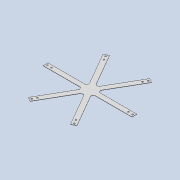
# Autodesk Inventor part: release_layer
Saved by Autodesk Inventor 2020 (Build 240168000, 168)
## iProperties
Created: 2021-10-03
Part Number: release_layer
Material: Generic
Document SubType Name: Modeling
Designer: Shuang Peng
Density: 1 g/cm^3
Appearance: Default
Author: Shuang Peng
Autodesk Inventor part; units mm, degrees
ref_plane "YZ Plane" through (0, 0, 0) normal (1, 0, 0) x (0, 1, 0)
ref_plane "XZ Plane" through (0, 0, 0) normal (0, 1, 0) x (-1, 0, 0)
ref_plane "XY Plane" through (0, 0, 0) normal (0, 0, 1) x (1, 0, 0)
sketch "Sketch1" plane through (0, 0, 0) normal (0, 1, 0) x (-1, 0, 0)
  line L0 (0, 0) -> (100, 0)
  line L1 (100, 0) -> (100, -100)
  line L2 (100, -100) -> (0, -100)
  line L3 (0, -100) -> (0, 0)
  dimension "d0" = 100
  dimension "d1" = 100
  constraints: 8 end point, 2 parallel, 1 horizontal, 1 perpendicular
  measures "d0" distance of L1.end L2.end
  measures "d1" distance of L0.end L1.end
extrude "Extrusion1" add sketch "Sketch1" along normal blind 0.2
sketch "Sketch2" plane through (0, 0.2, 0) normal (0, 1, 0) x (1, 0, 0)
  line L0 (-100, 0) -> (0, 0) projected
  line L1 (0, 0) -> (0, 50)
  line L2 (0, 50) -> (-50, 50)
  circle A0 centre (-50, 50) radius 6
  line L3 (-50, 50) -> (-77, 50)
  line L4 (-77, 48) -> (-77, 52)
  line L5 (-77, 52) -> (-50, 52)
  line L6 (-50, 52) -> (-50, 48)
  line L7 (-50, 48) -> (-77, 48)
  line L8 (-77, 48) -> (-50, 52) construction
  line L9 (-77, 52) -> (-50, 48) construction
  line L10 (-77, 50) -> (-82, 50)
  line L11 (-87, 48) -> (-87, 52)
  line L12 (-87, 52) -> (-77, 52)
  line L13 (-77, 52) -> (-77, 48)
  line L14 (-77, 48) -> (-87, 48)
  line L15 (-87, 48) -> (-77, 52) construction
  line L16 (-87, 52) -> (-77, 48) construction
  line L17 (-66.7679, 16.9571) -> (-70.2321, 18.9571)
  line L18 (-70.2321, 18.9571) -> (-65.2321, 27.6173)
  line L19 (-61.7679, 25.6173) -> (-66.7679, 16.9571)
  line L20 (-48.2679, 49) -> (-61.7679, 25.6173)
  line L21 (-65.2321, 27.6173) -> (-51.7321, 51)
  line L22 (-29.7679, 18.9571) -> (-33.2321, 16.9571)
  line L23 (-33.2321, 16.9571) -> (-38.2321, 25.6173)
  line L24 (-34.7679, 27.6173) -> (-29.7679, 18.9571)
  line L25 (-48.2679, 51) -> (-34.7679, 27.6173)
  line L26 (-38.2321, 25.6173) -> (-51.7321, 49)
  line L27 (-13, 52) -> (-13, 48)
  line L28 (-13, 48) -> (-23, 48)
  line L29 (-23, 52) -> (-13, 52)
  line L30 (-50, 52) -> (-23, 52)
  line L31 (-23, 48) -> (-50, 48)
  line L32 (-33.2321, 83.0429) -> (-29.7679, 81.0429)
  line L33 (-29.7679, 81.0429) -> (-34.7679, 72.3827)
  line L34 (-38.2321, 74.3827) -> (-33.2321, 83.0429)
  line L35 (-51.7321, 51) -> (-38.2321, 74.3827)
  line L36 (-34.7679, 72.3827) -> (-48.2679, 49)
  line L37 (-70.2321, 81.0429) -> (-66.7679, 83.0429)
  line L38 (-66.7679, 83.0429) -> (-61.7679, 74.3827)
  line L39 (-65.2321, 72.3827) -> (-70.2321, 81.0429)
  line L40 (-51.7321, 49) -> (-65.2321, 72.3827)
  line L41 (-61.7679, 74.3827) -> (-48.2679, 51)
  line L42 (-100, 0) -> (0, 0) projected
  line L43 (0, 0) -> (0, 100) projected
  line L44 (0, 100) -> (-100, 100) projected
  line L45 (-100, 100) -> (-100, 0) projected
  point P0 (-63.5, 50)
  point P1 (-44.3431, 48)
  point P2 (-45.4395, 46.101)
  point P3 (-48.9036, 44.101)
  point P4 (-51.0964, 44.101)
  point P5 (-54.5605, 46.101)
  point P6 (-55.6569, 48)
  point P7 (-55.6569, 52)
  point P8 (-54.5605, 53.899)
  point P9 (-51.0964, 55.899)
  point P10 (-48.9036, 55.899)
  point P11 (-45.4395, 53.899)
  point P12 (-44.3431, 52)
  dimension "d4" = 50
  dimension "d5" = 50
  dimension "d6" = 12
  dimension "d7" = 27
  dimension "d8" = 4
  dimension "d9" = 27
  dimension "d10" = 5
  dimension "d11" = 4
  dimension "d12" = 10
  dimension "d15" = 360
  constraints: 82 end point, 5 midpoint, 4 parallel, 3 perpendicular, 3 vertical, 2 horizontal, 1 centre point, 1 coincident, 79 other
  measures "d4" distance of L0.end L1.end
  measures "d5" distance of L1.end L2.end
  measures "d6" diameter of A0
  measures "d7" distance of L3.start L3.end
  measures "d8" distance of L4.start L4.end
  measures "d9" distance of L4.end L5.end
  measures "d10" distance of L3.end L10.end
  measures "d11" distance of L11.start L11.end
  measures "d12" distance of L11.end L12.end
extrude "Extrusion2" cut sketch "Sketch2" against normal blind 0.2
fillet "Fillet1" radius 1 12 edges at (-51.0964, 0.1, -44.101) (-48.9036, 0.1, -44.101) (-54.5605, 0.1, -46.101) (-55.6569, 0.1, -48) (-55.6569, 0.1, -52) (-54.5605, 0.1, -53.899) (-51.0964, 0.1, -55.899) (-48.9036, 0.1, -55.899) (-45.4395, 0.1, -53.899) (-44.3431, 0.1, -52) (-44.3431, 0.1, -48) (-45.4395, 0.1, -46.101)
sketch "Sketch3" plane through (0, 0.2, 0) normal (0, 1, 0) x (1, 0, 0)
  line L0 (-87, 48) -> (-56.3246, 48) projected
  line L1 (-66.7679, 16.9571) -> (-51.4302, 43.5228) projected
  arc A0 (-50.4836, 44.0195) -> (-51.4302, 43.5228) centre (-50.5642, 43.0228) ccw projected
  arc A1 (-50.4836, 44.0195) -> (-49.5164, 44.0195) centre (-50, 50) ccw projected
  arc A2 (-48.5698, 43.5228) -> (-49.5164, 44.0195) centre (-49.4358, 43.0228) ccw projected
  line L2 (-48.5698, 43.5228) -> (-33.2321, 16.9571) projected
  line L3 (-33.2321, 16.9571) -> (-29.7679, 18.9571) projected
  line L4 (-29.7679, 18.9571) -> (-45.1057, 45.5228) projected
  arc A3 (-45.0626, 46.5909) -> (-45.1057, 45.5228) centre (-44.2396, 46.0228) ccw projected
  arc A4 (-45.0626, 46.5909) -> (-44.579, 47.4286) centre (-50, 50) ccw projected
  arc A5 (-43.6754, 48) -> (-44.579, 47.4286) centre (-43.6754, 47) ccw projected
  line L5 (-43.6754, 48) -> (-13, 48) projected
  line L6 (-13, 48) -> (-13, 52) projected
  line L7 (-13, 52) -> (-43.6754, 52) projected
  arc A6 (-44.579, 52.5714) -> (-43.6754, 52) centre (-43.6754, 53) ccw projected
  arc A7 (-44.579, 52.5714) -> (-45.0626, 53.4091) centre (-50, 50) ccw projected
  arc A8 (-45.1057, 54.4772) -> (-45.0626, 53.4091) centre (-44.2396, 53.9772) ccw projected
  line L8 (-45.1057, 54.4772) -> (-29.7679, 81.0429) projected
  line L9 (-29.7679, 81.0429) -> (-33.2321, 83.0429) projected
  line L10 (-33.2321, 83.0429) -> (-48.5698, 56.4772) projected
  arc A9 (-49.5164, 55.9805) -> (-48.5698, 56.4772) centre (-49.4358, 56.9772) ccw projected
  arc A10 (-49.5164, 55.9805) -> (-50.4836, 55.9805) centre (-50, 50) ccw projected
  arc A11 (-51.4302, 56.4772) -> (-50.4836, 55.9805) centre (-50.5642, 56.9772) ccw projected
  line L11 (-51.4302, 56.4772) -> (-66.7679, 83.0429) projected
  line L12 (-66.7679, 83.0429) -> (-70.2321, 81.0429) projected
  line L13 (-70.2321, 81.0429) -> (-54.8943, 54.4772) projected
  arc A12 (-54.9374, 53.4091) -> (-54.8943, 54.4772) centre (-55.7604, 53.9772) ccw projected
  arc A13 (-54.9374, 53.4091) -> (-55.421, 52.5714) centre (-50, 50) ccw projected
  arc A14 (-56.3246, 52) -> (-55.421, 52.5714) centre (-56.3246, 53) ccw projected
  line L14 (-56.3246, 52) -> (-87, 52) projected
  line L15 (-87, 52) -> (-87, 48) projected
  line L16 (-87, 48) -> (-56.3246, 48) projected
  arc A15 (-55.421, 47.4286) -> (-56.3246, 48) centre (-56.3246, 47) ccw projected
  arc A16 (-55.421, 47.4286) -> (-54.9374, 46.5909) centre (-50, 50) ccw projected
  arc A17 (-54.8943, 45.5228) -> (-54.9374, 46.5909) centre (-55.7604, 46.0228) ccw projected
  line L17 (-54.8943, 45.5228) -> (-70.2321, 18.9571) projected
  line L18 (-70.2321, 18.9571) -> (-66.7679, 16.9571) projected
  line L19 (-50, 50) -> (-82, 50)
  line L20 (-82, 50) -> (-85.5, 50)
  circle A18 centre (-85.5, 50) radius 0.6
  circle A19 centre (-82, 50) radius 0.6
  point P0 (0, 0)
  dimension "d20" = 32
  dimension "d21" = 3.5
  dimension "d22" = 1.2
  dimension "d23" = 1.2
  constraints: 4 end point, 2 centre point, 2 coincident, 1 horizontal, 1 point on line
  measures "d20" distance of L19.start L19.end
  measures "d21" distance of L19.end L20.end
  measures "d22" diameter of A18
  measures "d23" diameter of A19
extrude "Extrusion3" cut sketch "Sketch3" against normal blind 0.2 contours A19 L20 L19 | L19 L20 A19 | A18
pattern_circular "Circular Pattern1" count 6 over 360 about axis through (-50, 0.2, -50) along (0, -1, 0) of "Extrusion3"
body "Solid1"
